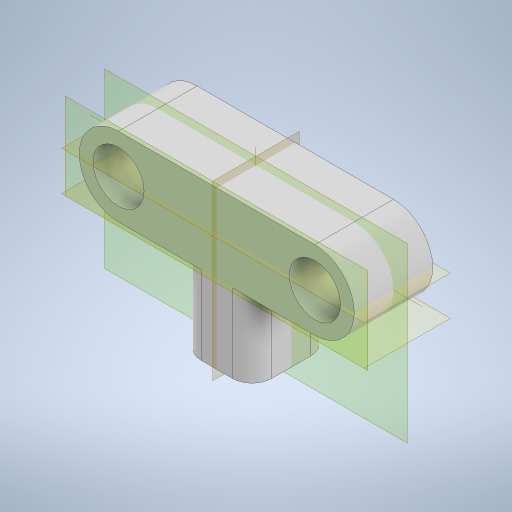
# Autodesk Inventor part: Schlitten1
Saved by Autodesk Inventor 2024 (Build 280153000, 153)
## iProperties
Created: 2025-06-04
Part Number: Schlitten1
Material: Generisch
Document SubType Name: Modeling
Designer: s0592566
Density: 1 g/cm^3
Appearance: Vorgabe
Author: s0592566
Autodesk Inventor part; units mm, degrees
sketch "Skizze1" plane through (0, 0, 0) normal (0, 1, 0) x (-1, 0, 0)
  line L0 (25, 10) -> (-25, 10)
  line L1 (-35, 0) -> (-35, 0)
  line L2 (-25, -10) -> (25, -10)
  line L3 (35, 0) -> (35, 0)
  line L4 (51.8995, 0) -> (-51.8995, 0) projected
  line L5 (0, -16.8995) -> (0, 16.8995) projected
  arc A0 (35, 8) -> (33, 10) centre (33, 8) ccw
  arc A1 (33, -10) -> (35, -8) centre (33, -8) ccw
  arc A2 (-33, 10) -> (-35, 8) centre (-33, 8) ccw
  arc A3 (-35, -8) -> (-33, -10) centre (-33, -8) ccw
  arc A4 (35, 0) -> (25, 10) centre (25, 0) ccw
  arc A5 (25, -10) -> (35, 0) centre (25, 0) ccw
  arc A6 (-25, 10) -> (-35, 0) centre (-25, 0) ccw
  arc A7 (-35, 0) -> (-25, -10) centre (-25, 0) ccw
  point P0 (0, 0)
  point P1 (-35, -10)
  point P2 (-35, 10)
  point P3 (35, -10)
  point P4 (-35, 0)
  dimension "d0" = 70
  dimension "d1" = 20
  dimension "d2" = 2
  dimension "d3" = 10
  constraints: 16 point on circle, 16 tangent, 14 point on line, 8 centre point, 8 end point, 6 equal radius, 2 parallel, 1 horizontal, 1 perpendicular, 2 other
  measures "d0" distance of point (35, -10) point (-35, -10)
  measures "d1" distance of point (-35, -10) point (-35, 10)
  measures "d2" radius of A0
  measures "d3" radius of A4
extrude "Extrusion1" add sketch "Skizze1" along normal mid plane 20
ref_plane "Arbeitsebene1" through (0, -10, 0) normal (0, 1, 0) x (-1, 0, 0)
sketch "Skizze3" plane through (0, -10, 0) normal (0, -1, 0) x (1, 0, 0)
  arc A0 (-25, 10) -> (-25, -10) centre (-25, 0) ccw projected
  arc A1 (25, -10) -> (25, 10) centre (25, 0) ccw projected
  point P0 (0, 0)
  constraints: 2 coincident
hole "Bohrung1" at (-25, -10, 0) at (25, -10, 0) direction (0, 1, 0) diameter 6.756 end through all counterbore diameter 13 counterbore depth 20
ref_plane "Arbeitsebene2" through (0, 0, -10) normal (0, 0, 1) x (1, 0, 0)
sketch "Skizze4" plane through (0, 0, -10) normal (0, 0, 1) x (1, 0, 0)
  line L0 (9, 10) -> (-9, 10)
  line L1 (-9, 10) -> (-9, -10)
  line L2 (-9, -10) -> (9, -10)
  line L3 (9, -10) -> (9, 10)
  line L4 (0, -26) -> (0, 16) projected
  line L5 (-49, 0) -> (49, 0) projected
  dimension "d15" = 18
  dimension "d16" = 20
  constraints: 8 end point, 2 parallel, 2 other
  measures "d15" distance of L2.end L1.end
  measures "d16" distance of L1.end L0.end
extrude "Extrusion2" add sketch "Skizze4" against normal blind 20
fillet "Rundung1" radius 5 4 edges at (-9, -10, -20) (9, -10, -20) (9, 10, -20) (-9, 10, -20)
